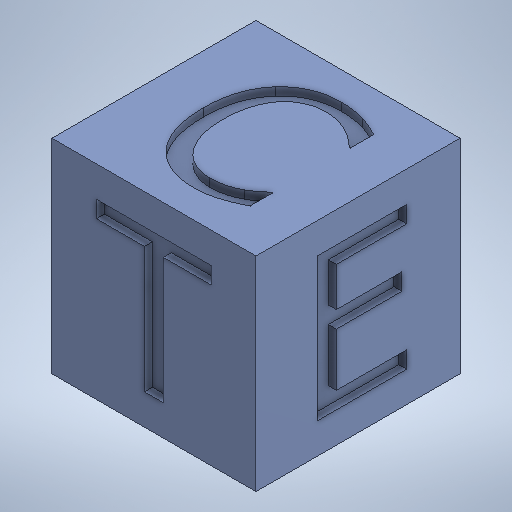
# Autodesk Inventor part: Cubo
Saved by Autodesk Inventor 2025.2 (Build 292293000, 293)
## iProperties
Created: 2025-01-18
Part Number: Cubo
Material: Rubber
Document SubType Name: Modeling
Designer: kenne
Density: 0.93 g/cm^3
Appearance: Rubber - Blue
Author: kenne
Autodesk Inventor part; units mm, degrees
ref_plane "YZ Plane" through (0, 0, 0) normal (1, 0, 0) x (0, 1, 0)
ref_plane "XZ Plane" through (0, 0, 0) normal (0, 1, 0) x (-1, 0, 0)
ref_plane "XY Plane" through (0, 0, 0) normal (0, 0, 1) x (1, 0, 0)
sketch "sqr_sketch" plane through (0, 0, 0) normal (1, 0, 0) x (0, 1, 0)
  line L0 (12.7, 12.7) -> (-12.7, 12.7)
  line L1 (-12.7, 12.7) -> (-12.7, -12.7)
  line L2 (-12.7, -12.7) -> (12.7, -12.7)
  line L3 (12.7, -12.7) -> (12.7, 12.7)
  line L4 (12.7, 12.7) -> (-12.7, -12.7) construction
  line L5 (-12.7, 12.7) -> (12.7, -12.7) construction
  point P0 (0, 0)
  dimension "d0" = 25.4
  constraints: 12 end point, 2 midpoint, 2 parallel, 2 perpendicular, 1 horizontal
  measures "d0" distance of L2.end L0.start
extrude "sqr_extrusion" add sketch "sqr_sketch" along normal mid plane 25.4
sketch "T_sketch" plane through (-12.7, -12.7, 12.7) normal (0, 0, 1) x (1, 0, 0)
  line L0 (5.5534, 21.59) -> (19.8466, 21.59) construction
  line L1 (19.8466, 21.59) -> (19.8466, 3.81) construction
  line L2 (19.8466, 3.81) -> (5.5534, 3.81) construction
  line L3 (5.5534, 3.81) -> (5.5534, 21.59) construction
  line L4 (12.7, 21.59) -> (12.7, 3.81) construction
  line L5 (11.5041, 3.81) -> (11.5041, 19.4864)
  line L6 (11.5041, 19.4864) -> (5.539, 19.4864)
  line L7 (5.539, 19.4864) -> (5.539, 21.59)
  line L8 (5.539, 21.59) -> (19.8322, 21.59)
  line L9 (19.8322, 21.59) -> (19.8322, 19.4864)
  line L10 (19.8322, 19.4864) -> (13.8671, 19.4864)
  line L11 (13.8671, 19.4864) -> (13.8671, 3.81)
  line L12 (13.8671, 3.81) -> (11.5041, 3.81)
  point P0 (12.7, 12.7)
  point P1 (12.7, 12.7)
  point P2 (5.5534, 12.7)
  point P3 (19.8466, 12.7)
  dimension "d17" = 17.78
  dimension "d18" = 14.2932
  constraints: 5 midpoint, 2 end point, 1 coincident, 1 horizontal alignment, 2 other
  measures "d17" distance of L2.end L0.start
  measures "d18" distance of L0.end L0.start
extrude "T_extrusion" cut sketch "T_sketch" against normal blind 1
sketch "E_sketch" plane through (12.7, 0, 0) normal (1, 0, 0) x (0, 0, -1)
  line L0 (-6.8584, 8.89) -> (6.8584, 8.89) construction
  line L1 (6.8584, 8.89) -> (6.8584, -8.89) construction
  line L2 (6.8584, -8.89) -> (-6.8584, -8.89) construction
  line L3 (-6.8584, -8.89) -> (-6.8584, 8.89) construction
  line L4 (0, 8.89) -> (0, -8.89) construction
  line L5 (-5.0574, -8.89) -> (-5.0574, 8.89)
  line L6 (-5.0574, 8.89) -> (6.0659, 8.89)
  line L7 (6.0659, 8.89) -> (6.0659, 6.7864)
  line L8 (6.0659, 6.7864) -> (-2.6944, 6.7864)
  line L9 (-2.6944, 6.7864) -> (-2.6944, 1.9163)
  line L10 (-2.6944, 1.9163) -> (5.4752, 1.9163)
  line L11 (5.4752, 1.9163) -> (5.4752, -0.1873)
  line L12 (5.4752, -0.1873) -> (-2.6944, -0.1873)
  line L13 (-2.6944, -0.1873) -> (-2.6944, -6.7864)
  line L14 (-2.6944, -6.7864) -> (6.0659, -6.7864)
  line L15 (6.0659, -6.7864) -> (6.0659, -8.89)
  line L16 (6.0659, -8.89) -> (-5.0574, -8.89)
  point P0 (0, 0)
  point P1 (0, 0)
  point P2 (-6.8584, 0)
  point P3 (6.8584, 0)
  dimension "d15" = 17.78
  dimension "d16" = 13.7168
  constraints: 5 midpoint, 2 end point, 1 coincident, 1 horizontal alignment, 2 other
  measures "d15" distance of L2.end L0.start
  measures "d16" distance of L0.end L0.start
extrude "E_extrusion" cut sketch "E_sketch" against normal blind 1
sketch "A_sketch" plane through (12.7, 12.7, -12.7) normal (0, 0, -1) x (-1, 0, 0)
  line L0 (5.2508, -3.81) -> (20.1492, -3.81) construction
  line L1 (20.1492, -3.81) -> (20.1492, -21.59) construction
  line L2 (20.1492, -21.59) -> (5.2508, -21.59) construction
  line L3 (5.2508, -21.59) -> (5.2508, -3.81) construction
  line L4 (12.7, -3.81) -> (12.7, -21.59) construction
  line L5 (5.1356, -21.59) -> (11.1295, -3.81)
  line L6 (11.1295, -3.81) -> (14.04, -3.81)
  line L7 (14.04, -3.81) -> (20.0339, -21.59)
  line L8 (20.0339, -21.59) -> (17.5412, -21.59)
  line L9 (17.5412, -21.59) -> (15.9275, -16.6191)
  line L10 (15.9275, -16.6191) -> (9.1411, -16.6191)
  line L11 (9.1411, -16.6191) -> (7.5274, -21.59)
  line L12 (7.5274, -21.59) -> (5.1356, -21.59)
  line L13 (15.2791, -14.6019) -> (12.5271, -6.2306)
  line L14 (12.5271, -6.2306) -> (9.7895, -14.6019)
  line L15 (9.7895, -14.6019) -> (15.2791, -14.6019)
  point P0 (12.7, -12.7)
  point P1 (5.2508, -12.7)
  point P2 (20.1492, -12.7)
  point P3 (12.7, -12.7)
  dimension "d19" = 17.78
  dimension "d20" = 14.8983
  constraints: 5 midpoint, 2 end point, 1 coincident, 1 horizontal alignment, 2 other
  measures "d19" distance of L2.end L0.start
  measures "d20" distance of L0.end L0.start
extrude "A_extrusion" cut sketch "A_sketch" against normal blind 1
sketch "R_sketch" plane through (-12.7, 0, 0) normal (-1, 0, 0) x (0, 0, 1)
  line L0 (-7.586, 8.89) -> (7.586, 8.89) construction
  line L1 (7.586, 8.89) -> (7.586, -8.89) construction
  line L2 (7.586, -8.89) -> (-7.586, -8.89) construction
  line L3 (-7.586, -8.89) -> (-7.586, 8.89) construction
  line L4 (0, 8.89) -> (0, -8.89) construction
  line L5 (7.9751, -8.89) -> (4.9061, -8.89)
  line L6 (4.9061, -8.89) -> (-0.7132, -1.8155)
  line L7 (-0.7132, -1.8155) -> (-3.422, -1.8155)
  line L8 (-3.422, -1.8155) -> (-3.422, -8.89)
  line L9 (-3.422, -8.89) -> (-5.785, -8.89)
  line L10 (-5.785, -8.89) -> (-5.785, 8.89)
  line L11 (-5.785, 8.89) -> (-1.2031, 8.89)
  spline S0 degree 2 poles (-1.2031, 8.89) (0.3242, 8.89) (2.3846, 8.5586) (3.3211, 7.9535) knots 0 0 0 1 2 2 2
  spline S1 degree 2 poles (3.3211, 7.9535) (4.2577, 7.3483) (5.3383, 5.4608) (5.3383, 4.0632) knots 0 0 0 1 2 2 2
  spline S2 degree 2 poles (5.3383, 4.0632) (5.3383, 2.118) (3.35, -0.5187) (1.6498, -1.1527) knots 0 0 0 1 2 2 2
  line L12 (1.6498, -1.1527) -> (7.9751, -8.89)
  spline S3 degree 2 poles (2.8745, 3.8759) (2.8745, 4.6539) (2.327, 5.8498) (1.7506, 6.2388) knots 0 0 0 1 2 2 2
  spline S4 degree 2 poles (1.7506, 6.2388) (1.2463, 6.5702) (-0.0937, 6.844) (-1.0734, 6.844) knots 0 0 0 1 2 2 2
  line L13 (-1.0734, 6.844) -> (-3.422, 6.844)
  line L14 (-3.422, 6.844) -> (-3.422, 0.1585)
  line L15 (-3.422, 0.1585) -> (-1.3472, 0.1585)
  spline S5 degree 2 poles (-1.3472, 0.1585) (-0.3242, 0.1585) (1.304, 0.5187) (1.8659, 1.0806) knots 0 0 0 1 2 2 2
  spline S6 degree 2 poles (1.8659, 1.0806) (2.3846, 1.5705) (2.8745, 2.9537) (2.8745, 3.8759) knots 0 0 0 1 2 2 2
  point P0 (0, 0)
  point P1 (0, 0)
  point P2 (-7.586, 0)
  point P3 (7.586, 0)
  dimension "d21" = 17.78
  dimension "d22" = 15.1721
  constraints: 5 midpoint, 2 end point, 1 coincident, 1 horizontal alignment, 2 other
  measures "d21" distance of L2.end L0.start
  measures "d22" distance of L0.end L0.start
extrude "R_extrusion" cut sketch "R_sketch" against normal blind 1
sketch "C_sketch" plane through (-12.7, 12.7, 12.7) normal (0, 1, 0) x (1, 0, 0)
  line L0 (5.3589, 21.907) -> (20.0411, 21.907) construction
  line L1 (20.0411, 21.907) -> (20.0411, 3.493) construction
  line L2 (20.0411, 3.493) -> (5.3589, 3.493) construction
  line L3 (5.3589, 3.493) -> (5.3589, 21.907) construction
  line L4 (12.7, 21.907) -> (12.7, 3.493) construction
  spline S0 degree 2 poles (14.1048, 3.493) (12.3758, 3.493) (9.4509, 4.6601) (8.3847, 5.8272) knots 0 0 0 1 2 2 2
  spline S1 degree 2 poles (8.3847, 5.8272) (7.3185, 6.9799) (6.1514, 10.4379) (6.1514, 12.6856) knots 0 0 0 1 2 2 2
  spline S2 degree 2 poles (6.1514, 12.6856) (6.1514, 14.9189) (7.2896, 18.2328) (8.3703, 19.4576) knots 0 0 0 1 2 2 2
  spline S3 degree 2 poles (8.3703, 19.4576) (9.4365, 20.6535) (12.347, 21.907) (14.148, 21.907) knots 0 0 0 1 2 2 2
  spline S4 degree 2 poles (14.148, 21.907) (15.0414, 21.907) (16.6119, 21.6476) (17.2747, 21.4459) knots 0 0 0 1 2 2 2
  spline S5 degree 2 poles (17.2747, 21.4459) (17.851, 21.2586) (19.0469, 20.7255) (19.6377, 20.4085) knots 0 0 0 1 2 2 2
  line L5 (19.6377, 20.4085) -> (19.6377, 17.5556)
  line L6 (19.6377, 17.5556) -> (19.4503, 17.5556)
  spline S6 degree 2 poles (19.4503, 17.5556) (19.1334, 17.8438) (18.1536, 18.6507) (17.4476, 19.0397) knots 0 0 0 1 2 2 2
  spline S7 degree 2 poles (17.4476, 19.0397) (16.7704, 19.4143) (15.171, 19.8898) (14.1336, 19.8898) knots 0 0 0 1 2 2 2
  spline S8 degree 2 poles (14.1336, 19.8898) (12.9954, 19.8898) (10.9638, 18.9533) (10.2001, 18.0599) knots 0 0 0 1 2 2 2
  spline S9 degree 2 poles (10.2001, 18.0599) (9.4509, 17.1522) (8.6152, 14.4002) (8.6152, 12.6856) knots 0 0 0 1 2 2 2
  spline S10 degree 2 poles (8.6152, 12.6856) (8.6152, 10.8557) (9.4941, 8.219) (10.2578, 7.3112) knots 0 0 0 1 2 2 2
  spline S11 degree 2 poles (10.2578, 7.3112) (11.007, 6.4323) (13.0098, 5.539) (14.1336, 5.539) knots 0 0 0 1 2 2 2
  spline S12 degree 2 poles (14.1336, 5.539) (15.1566, 5.539) (16.9001, 6.0433) (17.5773, 6.4179) knots 0 0 0 1 2 2 2
  spline S13 degree 2 poles (17.5773, 6.4179) (18.2256, 6.7925) (19.191, 7.5706) (19.4648, 7.8444) knots 0 0 0 1 2 2 2
  line L7 (19.4648, 7.8444) -> (19.6377, 7.8444)
  line L8 (19.6377, 7.8444) -> (19.6377, 5.0203)
  spline S14 degree 2 poles (19.6377, 5.0203) (19.0469, 4.7465) (18.0095, 4.2423) (17.2747, 4.0117) knots 0 0 0 1 2 2 2
  spline S15 degree 2 poles (17.2747, 4.0117) (16.4966, 3.7524) (15.171, 3.493) (14.1048, 3.493) knots 0 0 0 1 2 2 2
  point P0 (12.7, 12.7)
  point P1 (5.3589, 12.7)
  point P2 (20.0411, 12.7)
  point P3 (12.7, 12.7)
  dimension "d23" = 18.414
  dimension "d24" = 14.6822
  constraints: 5 midpoint, 2 end point, 1 coincident, 1 horizontal alignment, 2 other
  measures "d23" distance of L2.end L0.start
  measures "d24" distance of L0.end L0.start
extrude "C_extrusion" cut sketch "C_sketch" against normal blind 1
sketch "I_sketch" plane through (-12.7, -12.7, -12.7) normal (0, -1, 0) x (1, 0, 0)
  line L0 (8.1397, 21.59) -> (17.2603, 21.59) construction
  line L1 (17.2603, 21.59) -> (17.2603, 3.81) construction
  line L2 (17.2603, 3.81) -> (8.1397, 3.81) construction
  line L3 (8.1397, 3.81) -> (8.1397, 21.59) construction
  line L4 (12.7, 3.81) -> (12.7, 21.59) construction
  line L5 (16.1364, 3.81) -> (9.2492, 3.81)
  line L6 (9.2492, 3.81) -> (9.2492, 5.6255)
  line L7 (9.2492, 5.6255) -> (11.5113, 5.6255)
  line L8 (11.5113, 5.6255) -> (11.5113, 19.7745)
  line L9 (11.5113, 19.7745) -> (9.2492, 19.7745)
  line L10 (9.2492, 19.7745) -> (9.2492, 21.59)
  line L11 (9.2492, 21.59) -> (16.1364, 21.59)
  line L12 (16.1364, 21.59) -> (16.1364, 19.7745)
  line L13 (16.1364, 19.7745) -> (13.8743, 19.7745)
  line L14 (13.8743, 19.7745) -> (13.8743, 5.6255)
  line L15 (13.8743, 5.6255) -> (16.1364, 5.6255)
  line L16 (16.1364, 5.6255) -> (16.1364, 3.81)
  point P0 (12.7, 12.7)
  point P1 (17.2603, 12.7)
  point P2 (8.1397, 12.7)
  point P3 (12.7, 12.7)
  dimension "d25" = 17.78
  dimension "d26" = 9.1205
  constraints: 5 midpoint, 2 end point, 1 coincident, 1 horizontal alignment, 2 other
  measures "d25" distance of L0.end L1.end
  measures "d26" distance of L2.end L1.end
extrude "I_extrusion" cut sketch "I_sketch" against normal blind 1
equation "\"d1\" = d0"
